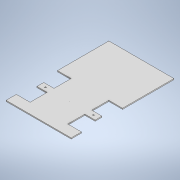
# Autodesk Inventor part: onderplaat v2
Saved by Autodesk Inventor 2022 (Build 260153000, 153)
## iProperties
Created: 2021-12-08
Part Number: onderplaat v2
Material: Generic
Document SubType Name: Modeling
Designer: keemi
Density: 1 g/cm^3
Appearance: Default
Author: keemi
Autodesk Inventor part; units mm, degrees
ref_plane "YZ Plane" through (0, 0, 0) normal (1, 0, 0) x (0, 1, 0)
ref_plane "XZ Plane" through (0, 0, 0) normal (0, 1, 0) x (-1, 0, 0)
ref_plane "XY Plane" through (0, 0, 0) normal (0, 0, 1) x (1, 0, 0)
sketch "Sketch1" plane through (0, 0, 0) normal (0, 1, 0) x (-1, 0, 0)
  line L0 (0, 0) -> (0, 300)
  line L1 (0, 300) -> (190, 300)
  line L2 (190, 300) -> (190, 0)
  line L3 (190, 0) -> (0, 0)
  line L4 (0, 300) -> (95, 300)
  line L5 (0, 300) -> (95, 300) construction
  line L6 (95, 300) -> (95, -51.2612)
  point P0 (95, 0)
  dimension "d0" = 300
  dimension "d1" = 190
  dimension "d2" = 90
  dimension "d3" = 300
  dimension "d4" = 90
  dimension "d23" = 95
  dimension "d24" = 0
  dimension "d25" = 90
  constraints: 14 end point, 2 collinear, 2 perpendicular, 1 horizontal, 1 vertical
  measures "d0" distance of L0.start L0.end
  measures "d1" distance of L0.end L1.end
  measures "d2" angle of L0 L1
  measures "d3" distance of L1.end L2.end
  measures "d4" angle of L1 L2
  measures "d23" distance of L0.end L4.end
  measures "d24" distance between parallel lines of L4 L5
  measures "d25" angle of L4 L6
extrude "Extrusion1" add sketch "Sketch1" along normal blind 3 contours L6 L1 L2 L3
sketch "Sketch2" plane through (0, 3, 0) normal (0, 1, 0) x (1, 0, 0)
  line L0 (-190, 0) -> (-190, -300) projected
  line L1 (-190, -300) -> (-190, -210)
  line L2 (-190, -210) -> (-190, -200)
  line L3 (-190, -200) -> (-190, -150)
  line L4 (-190, -210) -> (-190, -220)
  line L5 (-190, -150) -> (-150, -150)
  line L6 (-150, -150) -> (-150, -200)
  line L7 (-150, -200) -> (-190, -200)
  line L8 (-190, -200) -> (-190, -150)
  line L9 (-190, -220) -> (-150, -220)
  line L10 (-150, -220) -> (-150, -270)
  line L11 (-150, -270) -> (-190, -270)
  line L12 (-190, -270) -> (-190, -220)
  line L13 (-190, -220) -> (-180, -220)
  line L14 (-180, -220) -> (-180, -200)
  point P0 (0, 0)
  point P1 (-190, -270)
  dimension "d7" = 90
  dimension "d8" = 10
  dimension "d9" = 50
  dimension "d10" = 10
  dimension "d11" = 40
  dimension "d12" = 50
  dimension "d13" = 40
  dimension "d14" = 50
  dimension "d15" = 10
  constraints: 28 end point, 5 point on line, 4 parallel, 3 perpendicular, 2 horizontal, 1 midpoint
  measures "d7" distance of L0.end L1.end
  measures "d8" distance of L1.end L2.end
  measures "d9" distance of L2.end L3.end
  measures "d10" distance of L1.end L4.end
  measures "d11" distance of L6.end L7.end
  measures "d12" distance of L5.end L6.end
  measures "d13" distance of L10.end L11.end
  measures "d14" distance of L9.end L10.end
  measures "d15" distance of L4.end L13.end
extrude "Extrusion2" cut sketch "Sketch2" against normal blind 3
mirror "Mirror1" about plane through (-95, 0, 300) normal (1, 0, 0) of "Extrusion2", "Extrusion1"
sketch "Sketch4" plane through (0, 3, 0) normal (0, 1, 0) x (1, 0, 0)
  line L0 (-40, -200) -> (-10, -200) projected
  line L1 (-10, -200) -> (-10, -210)
  line L2 (-10, -200) -> (0, -200) construction
  line L3 (-10, -210) -> (-25, -210)
  line L4 (-180, -200) -> (-180, -210)
  line L5 (-180, -200) -> (-180, -220) projected
  line L6 (-180, -200) -> (-170, -200) construction
  line L7 (-180, -210) -> (-165, -210)
  circle A0 centre (-165, -210) radius 2
  circle A1 centre (-25, -210) radius 2
  point P0 (0, 0)
  dimension "d26" = 10
  dimension "d27" = 90
  dimension "d28" = 15
  dimension "d29" = 90
  dimension "d30" = 10
  dimension "d31" = 90
  dimension "d32" = 15
  dimension "d33" = 90
  dimension "d34" = 4
  dimension "d35" = 4
  constraints: 12 end point, 4 perpendicular, 2 centre point, 2 coincident, 2 horizontal, 1 collinear, 1 vertical
  measures "d26" distance of L0.end L1.end
  measures "d27" angle of L1 L2
  measures "d28" distance of L1.end L3.end
  measures "d29" angle of L1 L3
  measures "d30" distance of L4.start L4.end
  measures "d31" angle of L4 L6
  measures "d32" distance of L4.end L7.end
  measures "d33" angle of L7 L4
  measures "d34" diameter of A0
  measures "d35" diameter of A1
extrude "Extrusion4" cut sketch "Sketch4" against normal blind 10
sketch "Sketch5" plane through (0, 3, 0) normal (0, 1, 0) x (1, 0, 0)
  circle A0 centre (-165, -210) radius 2 projected
  line L0 (-165, -210) -> (-95, -210)
  circle A1 centre (-95, -210) radius 0.05
  point P0 (0, 0)
  dimension "d38" = 70
  dimension "d39" = 0.1
  constraints: 2 end point, 1 centre point, 1 coincident, 1 horizontal
  measures "d38" distance of L0.start L0.end
  measures "d39" diameter of A1
extrude "Extrusion5" cut sketch "Sketch5" against normal blind 10 contours A1
body "Solid1"
